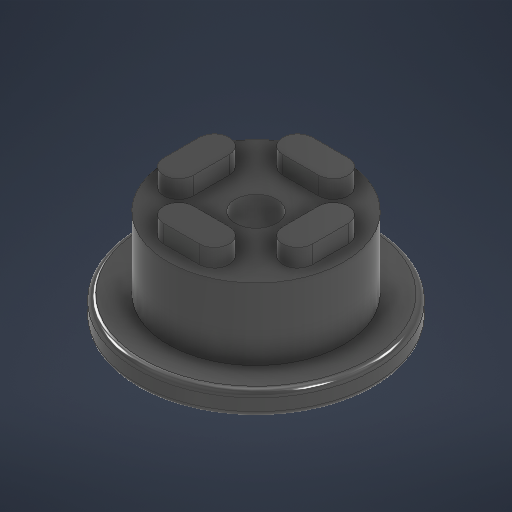
# Autodesk Inventor part: AxleCap
Saved by Autodesk Inventor 2026.2 (Build 302298010, 298A)
## iProperties
Created: 2026-02-18
Part Number: AxleCap
Material: Generic
Document SubType Name: Modeling
Designer: Liam
Density: 1 g/cm^3
Appearance: Default
Author: Liam
Autodesk Inventor part; units mm, degrees
ref_plane "YZ Plane" through (0, 0, 0) normal (1, 0, 0) x (0, 1, 0)
ref_plane "XZ Plane" through (0, 0, 0) normal (0, 1, 0) x (-1, 0, 0)
ref_plane "XY Plane" through (0, 0, 0) normal (0, 0, 1) x (1, 0, 0)
sketch "Sketch1" plane through (0, 0, 0) normal (0, 1, 0) x (-1, 0, 0)
  circle A0 centre (0, 0) radius 7.375
  circle A1 centre (0, 0) radius 1.75
  circle A2 centre (0, 0) radius 10
  circle A3 centre (0, 0) radius 3
  dimension "d0" = 14.75
  dimension "d1" = 3.5
  dimension "d2" = 20
  dimension "d7" = 6
  constraints: 4 centre point, 4 coincident
  measures "d0" diameter of A0
  measures "d1" diameter of A1
  measures "d2" diameter of A2
  measures "d7" diameter of A3
extrude "Extrusion1" add sketch "Sketch1" along normal blind 6 contours A0 | A3
extrude "Extrusion2" add sketch "Sketch1" against normal blind 2 contours A0 | A2
sketch "Sketch2" plane through (0, 6, 0) normal (0, 1, 0) x (1, 0, 0)
  line L0 (3.75, -2.75) -> (6.25, -2.75)
  line L1 (6.25, -2.75) -> (6.25, 2.75)
  line L2 (6.25, 2.75) -> (3.75, 2.75)
  line L3 (3.75, 2.75) -> (3.75, -2.75)
  line L4 (3.75, -2.75) -> (6.25, 2.75) construction
  line L5 (6.25, -2.75) -> (3.75, 2.75) construction
  line L6 (-2.75, 3.75) -> (2.75, 3.75)
  line L7 (2.75, 3.75) -> (2.75, 6.25)
  line L8 (2.75, 6.25) -> (-2.75, 6.25)
  line L9 (-2.75, 6.25) -> (-2.75, 3.75)
  line L10 (-3.75, -2.75) -> (-3.75, 2.75)
  line L11 (-3.75, 2.75) -> (-6.25, 2.75)
  line L12 (-6.25, 2.75) -> (-6.25, -2.75)
  line L13 (-6.25, -2.75) -> (-3.75, -2.75)
  line L14 (2.75, -3.75) -> (-2.75, -3.75)
  line L15 (-2.75, -3.75) -> (-2.75, -6.25)
  line L16 (-2.75, -6.25) -> (2.75, -6.25)
  line L17 (2.75, -6.25) -> (2.75, -3.75)
  point P0 (0, 0)
  point P1 (5, 0)
  dimension "d10" = 5.5
  dimension "d11" = 2.5
  dimension "d12" = 5
  dimension "d13" = 0
  dimension "d16" = 360
  constraints: 36 end point, 2 midpoint, 2 parallel, 1 horizontal, 1 perpendicular, 33 other
  measures "d10" distance of L2.end L0.start
  measures "d11" distance of L1.end L2.end
  measures "d12" distance of point (0, 0) point (5, 0)
  measures "d13" vertical distance of point (0, 0) point (5, 0)
extrude "Extrusion4" add sketch "Sketch2" along normal blind 1.5
fillet "Fillet1" radius 1.25 16 edges at (6.25, 6.75, -2.75) (3.75, 6.75, -2.75) (6.25, 6.75, 2.75) (3.75, 6.75, 2.75) (2.75, 6.75, 3.75) (2.75, 6.75, 6.25) (-2.75, 6.75, 6.25) (-2.75, 6.75, 3.75) (-3.75, 6.75, 2.75) (-6.25, 6.75, 2.75) (-6.25, 6.75, -2.75) (-3.75, 6.75, -2.75) (-2.75, 6.75, -6.25) (-2.75, 6.75, -3.75) (2.75, 6.75, -6.25) (2.75, 6.75, -3.75)
fillet "Fillet2" radius 0.5 3 edges at (10, -2, 0) (10, 0, 0) (3, -2, 0)
extrude "Extrusion5" cut sketch "Sketch1" along normal blind 3 contours A3
equation "\"d0\" = ShaftDiameter"
equation "\"d1\" = HoleDiameter"
equation "\"d2\" = CapDiameter"
equation "\"d3\" = ShaftLength"
equation "\"d5\" = CapLength"
equation "\"d18\" = TabLength"
equation "\"CapDiameter\" = 20"
equation "\"HoleDiameter\" = 3.5"
equation "\"ShaftLength\" = FEMUR_HEIGHT"
equation "\"CapLength\" = 2"
equation "\"HoleLength\" = 5"
equation "\"TabLength\" = 1.5"
equation "\"ShaftDiameter\" = 14.75"
equation "\"FEMUR_HEIGHT\" = 6"
body "Solid1"
